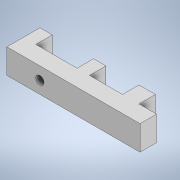
# Autodesk Inventor part: Elevator Side Holders
Saved by Autodesk Inventor 2022 (Build 260153000, 153)
## iProperties
Created: 2021-12-04
Part Number: Elevator Side Holders
Material: Generic
Document SubType Name: Modeling
Designer: merky
Density: 1 g/cm^3
Appearance: Default
Author: merky
Autodesk Inventor part; units mm, degrees
ref_plane "YZ Plane" through (0, 0, 0) normal (1, 0, 0) x (0, 1, 0)
ref_plane "XZ Plane" through (0, 0, 0) normal (0, 1, 0) x (-1, 0, 0)
ref_plane "XY Plane" through (0, 0, 0) normal (0, 0, 1) x (1, 0, 0)
sketch "Sketch1" plane through (0, 0, 0) normal (0, 1, 0) x (-1, 0, 0)
  line L0 (0, 0) -> (-30.48, 0)
  line L1 (-35.56, -10.16) -> (-2.54, -10.16)
  line L2 (-2.54, -10.16) -> (-2.54, -20.32)
  line L3 (-2.54, -20.32) -> (0, -20.32)
  line L4 (-35.56, -10.16) -> (-27.94, -10.16)
  line L5 (-27.94, -10.16) -> (-27.94, -20.32)
  line L6 (-27.94, -20.32) -> (-35.56, -20.32)
  line L7 (-35.56, -20.32) -> (-35.56, -10.16)
  line L8 (-2.54, -10.16) -> (-2.54, 0) construction
  line L9 (-27.94, -10.16) -> (-27.94, 0) construction
  line L10 (-27.94, -10.16) -> (-2.54, -10.16) construction
  line L11 (-2.54, -10.16) -> (-2.54, -60.96) construction
  line L12 (-2.54, -60.96) -> (-27.94, -60.96) construction
  line L13 (-27.94, -60.96) -> (-27.94, -10.16) construction
  line L14 (-66.04, -10.16) -> (-91.44, -10.16) construction
  line L15 (-91.44, -10.16) -> (-91.44, -60.96) construction
  line L16 (-91.44, -60.96) -> (-66.04, -60.96) construction
  line L17 (-66.04, -60.96) -> (-66.04, -10.16) construction
  line L18 (-30.48, 0) -> (-72.39, 0)
  line L19 (-72.39, 0) -> (-76.85, 0)
  line L20 (-76.85, 0) -> (-76.85, -10.16)
  line L21 (-76.85, -10.16) -> (-72.39, -10.16)
  line L22 (-55.88, -10.16) -> (-55.88, -20.32)
  line L23 (-55.88, -20.32) -> (-66.04, -20.32)
  line L24 (-66.04, -20.32) -> (-66.04, -10.16)
  line L25 (-72.39, -10.16) -> (-66.04, -10.16)
  line L26 (-55.88, -10.16) -> (-30.48, -10.16)
  line L27 (0, 0) -> (5.08, 0)
  line L28 (5.08, 0) -> (5.08, -17.78)
  line L29 (0, -20.32) -> (5.08, -20.32)
  line L30 (5.08, -20.32) -> (5.08, -17.78)
  point P0 (-66.04, 0)
  point P1 (-35.56, -10.16)
  dimension "d4" = 7.62
  dimension "d5" = 10.16
  dimension "d6" = 50.8
  dimension "d9" = 38.1
  dimension "d10" = 25.4
  dimension "d19" = 10.16
  dimension "d20" = 10.16
  constraints: 62 end point, 11 parallel, 8 horizontal, 8 perpendicular, 4 point on line
  measures "d4" distance of L5.end L6.end
  measures "d5" distance of L4.end L5.end
  measures "d6" distance of L1.end L11.end
  measures "d9" distance between parallel lines of L17 L13
  measures "d10" distance of L11.end L12.end
  measures "d19" distance of L22.start L22.end
  measures "d20" distance of L1.end L2.end
extrude "Extrusion1" add sketch "Sketch1" along normal blind 15.24
sketch "Sketch2" plane through (-5.08, 0, 0) normal (0, 0, 1) x (1, 0, 0)
  circle A0 centre (20.32, 7.62) radius 2.54
  point P0 (5.08, 0)
  dimension "d16" = 5.08
  constraints: 1 centre point, 1 coincident
  measures "d16" diameter of A0
extrude "Extrusion2" cut sketch "Sketch2" against normal through all
body "Solid1"
